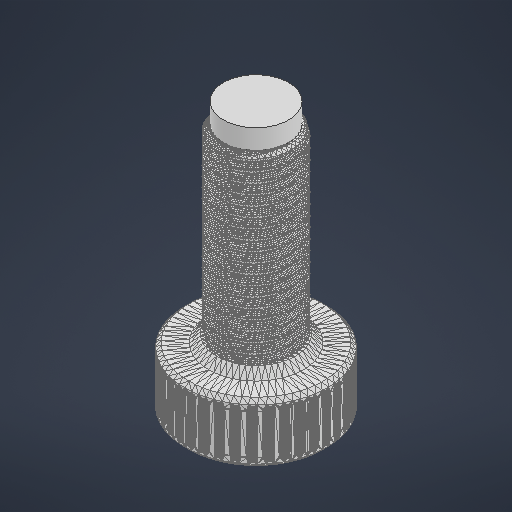
# Autodesk Inventor part: 111
Saved by Autodesk Inventor 2025 (Build 290162000, 162)
## iProperties
Created: 2026-04-24
Part Number: 111
Material: 常规
Document SubType Name: Modeling
Designer: XH
Density: 1 g/cm^3
Appearance: 默认
Author: XH
Autodesk Inventor part; units mm, degrees
ref_plane "YZ Plane" through (0, 0, 0) normal (1, 0, 0) x (0, 1, 0)
ref_plane "XZ Plane" through (0, 0, 0) normal (0, 1, 0) x (-1, 0, 0)
ref_plane "XY Plane" through (0, 0, 0) normal (0, 0, 1) x (1, 0, 0)
sketch "草图1" plane through (158.8794, 63, -173.2976) normal (0, 1, 0) x (-1, 0, 0)
  circle A0 centre (-2.6206, 8.2907) radius 8.2692 projected
  point P0 (158.8794, 173.2976)
extrude "拉伸1" add sketch "草图1" along normal blind 5
